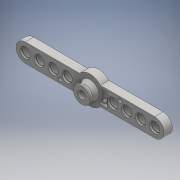
# Autodesk Inventor part: led-prop
Saved by Autodesk Inventor 2016 (Build 200138000, 138)
## iProperties
Created: 2016-11-01
Part Number: led-prop
Material: Generic
Document SubType Name: Modeling
Designer: Matt Ruffner
Density: 1 g/cm^3
Appearance: Default
Author: Matt Ruffner
Autodesk Inventor part; units mm, degrees
ref_plane "YZ Plane" through (0, 0, 0) normal (1, 0, 0) x (0, 1, 0)
ref_plane "XZ Plane" through (0, 0, 0) normal (0, 1, 0) x (-1, 0, 0)
ref_plane "XY Plane" through (0, 0, 0) normal (0, 0, 1) x (1, 0, 0)
sketch "Sketch1" plane through (0, 0, 0) normal (0, 1, 0) x (-1, 0, 0)
  circle A0 centre (24.5, 0) radius 5.05
  circle A1 centre (39.5, 0) radius 5.05
  circle A2 centre (54.5, 0) radius 5.05
  circle A3 centre (69.5, 0) radius 5.05
  circle A4 centre (-69.5, 0) radius 5.05
  circle A5 centre (-54.5, 0) radius 5.05
  circle A6 centre (-39.5, 0) radius 5.05
  circle A7 centre (-24.5, 0) radius 5.05
  line L0 (69.5, -10) -> (11.1803, -10)
  line L1 (69.5, 10) -> (11.1803, 10)
  arc A8 (69.5, -10) -> (69.5, 10) centre (69.5, 0) ccw
  line L2 (-69.5, -10) -> (-11.1803, -10)
  arc A9 (-69.5, 10) -> (-69.5, -10) centre (-69.5, 0) ccw
  line L3 (-69.5, 10) -> (-11.1803, 10)
  arc A10 (11.1803, 10) -> (-11.1803, 10) centre (0, 0) ccw
  arc A11 (-11.1803, -10) -> (11.1803, -10) centre (0, 0) ccw
  dimension "d1" = 10.1
  dimension "d2" = 10.1
  dimension "d3" = 10.1
  dimension "d4" = 10.1
  dimension "d5" = 24.5
  dimension "d6" = 15
  dimension "d7" = 15
  dimension "d8" = 15
  dimension "d11" = 360
  dimension "d16" = 360
  constraints: 12 centre point, 8 end point, 8 point on circle, 2 coincident, 2 horizontal, 34 other
  measures "d1" diameter of A0
  measures "d2" diameter of A1
  measures "d3" diameter of A2
  measures "d4" diameter of A3
  measures "d5" distance of A0.centre point (0, 0)
  measures "d6" distance of A1.centre A0.centre
  measures "d7" distance of A2.centre A1.centre
  measures "d8" distance of A3.centre A2.centre
extrude "Extrusion1" add sketch "Sketch1" along normal blind 9
sketch "Sketch2" plane through (0, 0, 0) normal (0, -1, 0) x (1, 0, 0)
  circle A0 centre (-69.5, 0) radius 5.05 projected
  circle A1 centre (-54.5, 0) radius 5.05 projected
  circle A2 centre (-39.5, 0) radius 5.05 projected
  circle A3 centre (-24.5, 0) radius 5.05 projected
  circle A4 centre (24.5, 0) radius 5.05 projected
  circle A5 centre (39.5, 0) radius 5.05 projected
  circle A6 centre (54.5, 0) radius 5.05 projected
  circle A7 centre (69.5, 0) radius 5.05 projected
  circle A8 centre (-69.5, 0) radius 5.6
  circle A9 centre (-54.5, 0) radius 5.6
  circle A10 centre (-39.5, 0) radius 5.6
  circle A11 centre (-24.5, 0) radius 5.6
  circle A12 centre (24.5, 0) radius 5.6
  circle A13 centre (39.5, 0) radius 5.6
  circle A14 centre (54.5, 0) radius 5.6
  circle A15 centre (69.5, 0) radius 5.6
  point P0 (0, 0)
  dimension "d20" = 11.2
  dimension "d21" = 11.2
  dimension "d22" = 11.2
  dimension "d23" = 11.2
  dimension "d24" = 11.2
  dimension "d25" = 11.2
  dimension "d26" = 11.2
  dimension "d27" = 11.2
  constraints: 8 centre point, 8 coincident
  measures "d20" diameter of A8
  measures "d21" diameter of A9
  measures "d22" diameter of A10
  measures "d23" diameter of A11
  measures "d24" diameter of A12
  measures "d25" diameter of A13
  measures "d26" diameter of A14
  measures "d27" diameter of A15
extrude "Extrusion2" cut sketch "Sketch2" against normal blind 2
sketch "Sketch5" plane through (0, 0, 0) normal (0, -1, 0) x (1, 0, 0)
  line L0 (9.9999, 7.45) -> (18.4999, 7.45)
  line L1 (18.4999, 7.45) -> (18.4999, -7.45)
  line L2 (18.4999, -7.45) -> (9.9999, -7.45)
  line L3 (9.9999, -7.45) -> (9.9999, 7.45)
  line L4 (69.5, 10) -> (11.1803, 10) projected
  circle A0 centre (14.1999, -4.5) radius 1.55
  point P0 (0, 0)
  point P1 (9.7499, -0.0369)
  dimension "d52" = 8.5
  dimension "d53" = 14.9
  dimension "d54" = 2.55
  dimension "d55" = 0.25
  dimension "d56" = 3.1
  dimension "d57" = 2.95
  constraints: 8 end point, 2 parallel, 1 centre point, 1 horizontal, 1 perpendicular
  measures "d52" distance of L1.end L2.end
  measures "d53" distance of L0.end L1.end
  measures "d54" distance between parallel lines of L4 L0
  measures "d55" distance from line of point (9.75, -0.037) L3
  measures "d56" diameter of A0
  measures "d57" distance from line of L2 A0.centre
extrude "Extrusion4" cut sketch "Sketch5" against normal blind 3.5
sketch "Sketch6" plane through (0, 0, 0) normal (0, -1, 0) x (1, 0, 0)
  circle A0 centre (32, 6) radius 2
  circle A1 centre (24.5, 0) radius 5.05 projected
  circle A2 centre (-32, -6) radius 2
  circle A3 centre (-24.5, 0) radius 5.05 projected
  point P0 (0, 0)
  dimension "d60" = 4
  dimension "d61" = 7.5
  dimension "d62" = 6
  dimension "d63" = 4
  dimension "d64" = 7.5
  dimension "d65" = 6
  constraints: 2 centre point
  measures "d60" diameter of A0
  measures "d61" horizontal distance of A1.centre A0.centre
  measures "d62" vertical distance of A1.centre A0.centre
  measures "d63" diameter of A2
  measures "d64" horizontal distance of A3.centre A2.centre
  measures "d65" vertical distance of A3.centre A2.centre
extrude "Extrusion5" cut sketch "Sketch6" against normal through all contours A0 | A2
sketch "Sketch8" plane through (0, 0, 0) normal (0, -1, 0) x (1, 0, 0)
  point P0 (0, 0)
  point P1 (0, 0)
  constraints: 1 coincident
ref_plane "Work Plane1" through (-0.0001, 0, 7.45) normal (1, 0, 0) x (0, 0, -1)
sketch "Sketch9" plane through (-0.0001, 0, 7.45) normal (1, 0, 0) x (0, 0, -1)
  line L0 (7.45, 0) -> (-2.3, 0)
  line L1 (-2.55, 0) -> (17.45, 0) projected
  line L2 (7.45, 0) -> (7.45, -9)
  line L3 (7.45, -9) -> (-2.3, -9)
  line L4 (-2.3, -9) -> (0.45, -4.5)
  line L5 (-2.3, 0) -> (0.45, -4.5)
  dimension "d74" = 9
  constraints: 10 end point, 1 perpendicular, 1 point on line, 1 vertical
  measures "d74" distance of L0.start L2.end
revolve "Revolution1" add sketch "Sketch9" angle 360 about axis through (-0.0001, 0, 0) along (0, -1, 0)
sketch "Sketch10" plane through (-0.0001, -9, 0) normal (0, -1, 0) x (1, 0, 0)
  circle A0 centre (0.0001, 0) radius 4.1
  dimension "d76" = 8.2
  constraints: 1 centre point, 1 coincident
  measures "d76" diameter of A0
extrude "Extrusion6" cut sketch "Sketch10" against normal through all
chamfer "Chamfer1" distance 1 angle 45 1 edges at (-0.0001, -9, -9.75)
body "Solid1"
